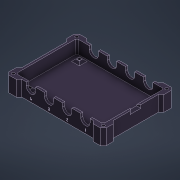
# Autodesk Inventor part: Case
Saved by Autodesk Inventor 2021.3 (Build 253353000, 353)
## iProperties
Created: 2022-02-15
Part Number: Case
Material: Generic
Document SubType Name: Modeling
Designer: Alex
Density: 1 g/cm^3
Appearance: Default
Author: Alex
Autodesk Inventor part; units mm, degrees
ref_plane "YZ Plane" through (0, 0, 0) normal (1, 0, 0) x (0, 1, 0)
ref_plane "XZ Plane" through (0, 0, 0) normal (0, 1, 0) x (-1, 0, 0)
ref_plane "XY Plane" through (0, 0, 0) normal (0, 0, 1) x (1, 0, 0)
sketch "Sketch1" plane through (0, 0, 0) normal (0, 1, 0) x (-1, 0, 0)
  line L0 (0, -45.5) -> (-50, -45.5)
  line L1 (-50, -45.5) -> (-54, -49.5)
  line L2 (-54, -49.5) -> (-64, -49.5)
  line L3 (-64, -49.5) -> (-68, -45.5)
  line L4 (-68, -45.5) -> (-68, -35.5)
  line L5 (-68, -35.5) -> (-64, -31.5)
  line L6 (-64, -31.5) -> (-64, 0)
  line L7 (0, 0) -> (0, -45.5) construction
  line L8 (0, 0) -> (-64, 0) construction
  line L9 (0, -45.5) -> (50, -45.5)
  line L10 (50, -45.5) -> (54, -49.5)
  line L11 (54, -49.5) -> (64, -49.5)
  line L12 (64, -49.5) -> (68, -45.5)
  line L13 (68, -45.5) -> (68, -35.5)
  line L14 (68, -35.5) -> (64, -31.5)
  line L15 (64, -31.5) -> (64, 0)
  line L16 (0, 0) -> (64, 0) construction
  line L17 (0, 45.5) -> (-50, 45.5)
  line L18 (-50, 45.5) -> (-54, 49.5)
  line L19 (-54, 49.5) -> (-64, 49.5)
  line L20 (-64, 49.5) -> (-68, 45.5)
  line L21 (-68, 45.5) -> (-68, 35.5)
  line L22 (-68, 35.5) -> (-64, 31.5)
  line L23 (-64, 31.5) -> (-64, 0)
  line L24 (0, 0) -> (0, 45.5) construction
  line L25 (0, 45.5) -> (50, 45.5)
  line L26 (50, 45.5) -> (54, 49.5)
  line L27 (54, 49.5) -> (64, 49.5)
  line L28 (64, 49.5) -> (68, 45.5)
  line L29 (68, 45.5) -> (68, 35.5)
  line L30 (68, 35.5) -> (64, 31.5)
  line L31 (64, 31.5) -> (64, 0)
  dimension "d6" = 100
  dimension "d7" = 10
  dimension "d10" = 135
  dimension "d11" = 4
  dimension "d22" = 91
  constraints: 64 end point, 20 symmetric about line, 3 perpendicular, 2 horizontal, 2 horizontal alignment, 2 vertical, 2 vertical alignment
  measures "d6" diameter of L0.end L7
  measures "d7" distance of L1.end L2.end
  measures "d10" angle of L0 L1
  measures "d11" distance from line of L3.end L2
  measures "d22" distance between parallel lines of L17 L0
extrude "Extrusion1" add sketch "Sketch1" along normal blind 3
sketch "Sketch2" plane through (0, 3, 0) normal (0, 1, 0) x (1, 0, 0)
  line L0 (-61, 42.5) -> (61, 42.5)
  line L1 (61, 42.5) -> (61, -42.5)
  line L2 (61, -42.5) -> (-61, -42.5)
  line L3 (-61, -42.5) -> (-61, 42.5)
  line L4 (-54, 49.5) -> (-64, 49.5) projected
  line L5 (-64, 49.5) -> (-68, 45.5) projected
  line L6 (-68, 45.5) -> (-68, 35.5) projected
  line L7 (-68, 35.5) -> (-64, 31.5) projected
  line L8 (-64, 31.5) -> (-64, -31.5) projected
  line L9 (-64, -31.5) -> (-68, -35.5) projected
  line L10 (-68, -35.5) -> (-68, -45.5) projected
  line L11 (-68, -45.5) -> (-64, -49.5) projected
  line L12 (-64, -49.5) -> (-54, -49.5) projected
  line L13 (-54, -49.5) -> (-50, -45.5) projected
  line L14 (-50, -45.5) -> (50, -45.5) projected
  line L15 (50, -45.5) -> (54, -49.5) projected
  line L16 (54, -49.5) -> (64, -49.5) projected
  line L17 (64, -49.5) -> (68, -45.5) projected
  line L18 (68, -45.5) -> (68, -35.5) projected
  line L19 (68, -35.5) -> (64, -31.5) projected
  line L20 (64, -31.5) -> (64, 31.5) projected
  line L21 (64, 31.5) -> (68, 35.5) projected
  line L22 (68, 35.5) -> (68, 45.5) projected
  line L23 (68, 45.5) -> (64, 49.5) projected
  line L24 (64, 49.5) -> (54, 49.5) projected
  line L25 (54, 49.5) -> (50, 45.5) projected
  line L26 (50, 45.5) -> (-50, 45.5) projected
  line L27 (-50, 45.5) -> (-54, 49.5) projected
  line L28 (-49.9676, 41.5746) -> (66.2374, 41.5746) construction
  line L29 (66.2374, 41.5746) -> (66.2374, -40.9754) construction
  line L30 (66.2374, -40.9754) -> (-49.9676, -40.9754) construction
  line L31 (-49.9676, -40.9754) -> (-49.9676, 41.5746) construction
  point P0 (0, 0)
  point P1 (-61, 0)
  point P2 (0, 42.5)
  dimension "d14" = 3
  dimension "d15" = 3
  dimension "d16" = 116.205
  dimension "d17" = 82.55
  constraints: 16 end point, 3 horizontal, 3 vertical, 2 midpoint, 1 horizontal alignment, 1 vertical alignment
  measures "d14" distance between parallel lines of L26 L0
  measures "d15" distance between parallel lines of L8 L3
  measures "d16" distance of L28.start L28.end
  measures "d17" distance of L30.end L28.start
extrude "Extrusion2" add sketch "Sketch2" along normal blind 18.5
sketch "Sketch4" plane through (0, 3, 0) normal (0, 1, 0) x (1, 0, 0)
  line L0 (-56.205, 41.275) -> (60, 41.275) construction
  line L1 (60, 41.275) -> (60, -41.275) construction
  line L2 (60, -41.275) -> (-56.205, -41.275) construction
  line L3 (-56.205, -41.275) -> (-56.205, 41.275) construction
  line L4 (-61, 42.5) -> (-61, -42.5) construction
  line L5 (-61, -42.5) -> (61, -42.5) construction
  line L6 (61, -42.5) -> (61, 42.5) construction
  line L7 (61, 42.5) -> (-61, 42.5) construction
  line L8 (-64, 49.5) -> (-68, 45.5) construction
  line L9 (-68, 45.5) -> (-68, 35.5) construction
  line L10 (-68, 35.5) -> (-64, 31.5) construction
  line L11 (-64, 31.5) -> (-64, -31.5) construction
  line L12 (-64, -31.5) -> (-68, -35.5) construction
  line L13 (-68, -35.5) -> (-68, -45.5) construction
  line L14 (-68, -45.5) -> (-64, -49.5) construction
  line L15 (-64, -49.5) -> (-54, -49.5) construction
  line L16 (-54, -49.5) -> (-50, -45.5) construction
  line L17 (-50, -45.5) -> (50, -45.5) construction
  line L18 (50, -45.5) -> (54, -49.5) construction
  line L19 (54, -49.5) -> (64, -49.5) construction
  line L20 (64, -49.5) -> (68, -45.5) construction
  line L21 (68, -45.5) -> (68, -35.5) construction
  line L22 (68, -35.5) -> (64, -31.5) construction
  line L23 (64, -31.5) -> (64, 31.5) construction
  line L24 (64, 31.5) -> (68, 35.5) construction
  line L25 (68, 35.5) -> (68, 45.5) construction
  line L26 (68, 45.5) -> (64, 49.5) construction
  line L27 (64, 49.5) -> (54, 49.5) construction
  line L28 (54, 49.5) -> (50, 45.5) construction
  line L29 (50, 45.5) -> (-50, 45.5) construction
  line L30 (-50, 45.5) -> (-54, 49.5) construction
  line L31 (-54, 49.5) -> (-64, 49.5) construction
  line L32 (-61, 42.5) -> (61, 42.5) construction
  line L33 (61, 42.5) -> (61, -42.5) construction
  line L34 (61, -42.5) -> (-61, -42.5) construction
  line L35 (-61, -42.5) -> (-61, 42.5) construction
  line L36 (-52.355, 37.425) -> (-47.355, 37.425)
  line L37 (-47.355, 37.425) -> (-47.355, 32.425)
  line L38 (-47.355, 32.425) -> (-52.355, 32.425)
  line L39 (-52.355, 32.425) -> (-52.355, 37.425)
  line L40 (-52.355, 37.425) -> (-47.355, 32.425) construction
  line L41 (-47.355, 37.425) -> (-52.355, 32.425) construction
  line L42 (-52.355, -32.425) -> (-52.355, -37.425)
  line L43 (-52.355, -37.425) -> (-47.355, -37.425)
  line L44 (-47.355, -37.425) -> (-47.355, -32.425)
  line L45 (-47.355, -32.425) -> (-52.355, -32.425)
  line L46 (-52.355, -32.425) -> (-47.355, -37.425) construction
  line L47 (-52.355, -37.425) -> (-47.355, -32.425) construction
  line L48 (51.15, 37.425) -> (56.15, 37.425)
  line L49 (56.15, 37.425) -> (56.15, 32.425)
  line L50 (56.15, 32.425) -> (51.15, 32.425)
  line L51 (51.15, 32.425) -> (51.15, 37.425)
  line L52 (51.15, 37.425) -> (56.15, 32.425) construction
  line L53 (56.15, 37.425) -> (51.15, 32.425) construction
  line L54 (51.15, -32.425) -> (56.15, -32.425)
  line L55 (56.15, -32.425) -> (56.15, -37.425)
  line L56 (56.15, -37.425) -> (51.15, -37.425)
  line L57 (51.15, -37.425) -> (51.15, -32.425)
  line L58 (51.15, -32.425) -> (56.15, -37.425) construction
  line L59 (56.15, -32.425) -> (51.15, -37.425) construction
  point P0 (-61, 0)
  point P1 (-56.205, 0)
  point P2 (-49.855, 34.925)
  point P3 (-49.855, -34.925)
  point P4 (53.65, 34.925)
  point P5 (53.65, -34.925)
  point P6 (-49.855, 34.925)
  point P7 (53.65, 34.925)
  point P8 (53.65, -34.925)
  point P9 (-49.855, -34.925)
  point P10 (-49.855, 34.925)
  point P11 (-49.855, -34.925)
  point P12 (53.65, -34.925)
  point P13 (53.65, 34.925)
  dimension "d20" = 116.205
  dimension "d21" = 82.55
  dimension "d23" = 6.35
  dimension "d24" = 6.35
  dimension "d25" = 6.35
  dimension "d26" = 6.35
  dimension "d27" = 5
  dimension "d28" = 1
  constraints: 56 end point, 18 midpoint, 10 horizontal, 10 vertical, 6 equal length, 3 horizontal alignment, 2 vertical alignment, 1 point on line
  measures "d20" distance of L0.start L0.end
  measures "d21" distance of L2.end L0.start
  measures "d23" distance from line of point (-49.855, 34.925) L3
  measures "d24" distance from line of point (53.65, 34.925) L1
  measures "d25" distance from line of L0 point (-49.855, 34.925)
  measures "d26" distance from line of point (-49.855, -34.925) L2
  measures "d27" distance of L36.end L37.end
  measures "d28" distance between parallel lines of L1 L6
extrude "Extrusion3" add sketch "Sketch4" along normal blind 3
chamfer "Chamfer1" distance 3 angle 45 16 edges at (-49.855, 3, -32.425) (-47.355, 3, -34.925) (-49.855, 3, -37.425) (-52.355, 3, -34.925) (53.65, 3, -32.425) (56.15, 3, -34.925) (53.65, 3, -37.425) (51.15, 3, -34.925) (53.65, 3, 32.425) (51.15, 3, 34.925) (53.65, 3, 37.425) (56.15, 3, 34.925) (-52.355, 3, 34.925) (-49.855, 3, 32.425) (-47.355, 3, 34.925) (-49.855, 3, 37.425)
sketch "Sketch5" plane through (0, 6, 0) normal (0, 1, 0) x (1, 0, 0)
  line L0 (48.15, -29.425) -> (48.15, -40.425) construction
  line L1 (59.15, -29.425) -> (48.15, -29.425) construction
  line L2 (59.15, -40.425) -> (59.15, -29.425) construction
  line L3 (48.15, -40.425) -> (59.15, -40.425) construction
  line L4 (-44.355, 29.425) -> (-44.355, 40.425) construction
  line L5 (-55.355, 29.425) -> (-44.355, 29.425) construction
  line L6 (-55.355, 40.425) -> (-55.355, 29.425) construction
  line L7 (-44.355, 40.425) -> (-55.355, 40.425) construction
  line L8 (-61, 42.5) -> (-61, -42.5) construction
  line L9 (-61, -42.5) -> (61, -42.5) construction
  line L10 (61, -42.5) -> (61, 42.5) construction
  line L11 (61, 42.5) -> (-61, 42.5) construction
  line L12 (59.15, 29.425) -> (59.15, 40.425) construction
  line L13 (48.15, 29.425) -> (59.15, 29.425) construction
  line L14 (48.15, 40.425) -> (48.15, 29.425) construction
  line L15 (59.15, 40.425) -> (48.15, 40.425) construction
  line L16 (-55.355, -29.425) -> (-55.355, -40.425) construction
  line L17 (-44.355, -29.425) -> (-55.355, -29.425) construction
  line L18 (-44.355, -40.425) -> (-44.355, -29.425) construction
  line L19 (-55.355, -40.425) -> (-44.355, -40.425) construction
  line L20 (-52.355, 32.425) -> (-47.355, 32.425) construction
  line L21 (-47.355, 32.425) -> (-47.355, 37.425) construction
  line L22 (-47.355, 37.425) -> (-52.355, 37.425) construction
  line L23 (-52.355, 37.425) -> (-52.355, 32.425) construction
  line L24 (51.15, 32.425) -> (56.15, 32.425) construction
  line L25 (56.15, 32.425) -> (56.15, 37.425) construction
  line L26 (56.15, 37.425) -> (51.15, 37.425) construction
  line L27 (51.15, 37.425) -> (51.15, 32.425) construction
  line L28 (51.15, -37.425) -> (56.15, -37.425) construction
  line L29 (56.15, -37.425) -> (56.15, -32.425) construction
  line L30 (56.15, -32.425) -> (51.15, -32.425) construction
  line L31 (51.15, -32.425) -> (51.15, -37.425) construction
  line L32 (-52.355, -37.425) -> (-47.355, -37.425) construction
  line L33 (-47.355, -37.425) -> (-47.355, -32.425) construction
  line L34 (-47.355, -32.425) -> (-52.355, -32.425) construction
  line L35 (-52.355, -32.425) -> (-52.355, -37.425) construction
  point P0 (0, 0)
  point P1 (-49.855, 34.925)
  point P2 (53.65, 34.925)
  point P3 (53.65, -34.925)
  point P4 (-49.855, -34.925)
  point P5 (-49.855, 37.425)
  point P6 (53.65, 37.425)
  point P7 (53.65, -32.425)
  point P8 (-49.855, -32.425)
  point P9 (-47.355, -34.925)
  point P10 (-47.355, 34.925)
  point P11 (56.15, 34.925)
  point P12 (56.15, -34.925)
  constraints: 8 midpoint, 4 horizontal alignment, 4 vertical alignment
hole "Hole1" at (-49.855, 6, -34.925) at (53.65, 6, -34.925) at (53.65, 6, 34.925) at (-49.855, 6, 34.925) direction (0, -1, 0) diameter 4 depth 5
sketch "Sketch6" plane through (-50, 0, 45.5) normal (0, 0, 1) x (1, 0, 0)
  line L0 (110, 3) -> (-6.205, 3) construction
  line L1 (-5.355, 3) -> (-2.355, 6) construction
  line L2 (2.645, 6) -> (5.645, 3) construction
  line L3 (-2.355, 6) -> (2.645, 6) construction
  line L4 (98.15, 3) -> (109.15, 3) construction
  line L5 (106.15, 6) -> (109.15, 3) construction
  line L6 (101.15, 6) -> (106.15, 6) construction
  line L7 (98.15, 3) -> (101.15, 6) construction
  line L8 (106.15, 6) -> (109.15, 3) construction
  line L9 (101.15, 6) -> (106.15, 6) construction
  line L10 (98.15, 3) -> (109.15, 3) construction
  line L11 (106.15, 6) -> (109.15, 3) construction
  line L12 (101.15, 6) -> (106.15, 6) construction
  line L13 (98.15, 3) -> (101.15, 6) construction
  line L14 (-1.855, 6) -> (2.145, 6) construction
  line L15 (-6.205, 7.65) -> (110, 7.65) construction
  line L16 (110, 7.65) -> (110, 6) construction
  line L17 (110, 6) -> (-6.205, 6) construction
  line L18 (-6.205, 6) -> (-6.205, 7.65) construction
  arc A0 (6.345, 16.4) -> (19.345, 16.4) centre (12.845, 16.4) ccw
  line L19 (0, 0) -> (0, 21.5) construction
  line L20 (0, 21.5) -> (100, 21.5) construction
  line L21 (100, 0) -> (100, 21.5) construction
  line L22 (0, 0) -> (100, 0) construction
  line L23 (19.345, 16.4) -> (19.345, 21.5)
  line L24 (6.345, 16.4) -> (6.345, 21.5)
  line L25 (6.345, 21.5) -> (19.345, 21.5)
  arc A1 (19.345, 16.4) -> (6.345, 16.4) centre (12.845, 16.4) ccw construction
  arc A2 (31.745, 16.4) -> (44.745, 16.4) centre (38.245, 16.4) ccw
  arc A3 (44.745, 16.4) -> (31.745, 16.4) centre (38.245, 16.4) ccw construction
  line L26 (31.745, 16.4) -> (31.745, 21.5)
  line L27 (44.745, 16.4) -> (44.745, 21.5)
  line L28 (31.745, 21.5) -> (44.745, 21.5)
  arc A4 (57.145, 16.4) -> (70.145, 16.4) centre (63.645, 16.4) ccw
  arc A5 (70.145, 16.4) -> (57.145, 16.4) centre (63.645, 16.4) ccw construction
  line L29 (57.145, 16.4) -> (57.145, 21.5)
  line L30 (70.145, 16.4) -> (70.145, 21.5)
  line L31 (57.145, 21.5) -> (70.145, 21.5)
  arc A6 (82.545, 16.4) -> (95.545, 16.4) centre (89.045, 16.4) ccw
  arc A7 (95.545, 16.4) -> (82.545, 16.4) centre (89.045, 16.4) ccw construction
  line L32 (82.545, 16.4) -> (82.545, 21.5)
  line L33 (95.545, 16.4) -> (95.545, 21.5)
  line L34 (82.545, 21.5) -> (95.545, 21.5)
  point P0 (50, 0)
  point P1 (0.145, 3)
  dimension "d41" = 1.65
  dimension "d42" = 116.205
  dimension "d43" = 6.35
  dimension "d44" = 13
  dimension "d46" = 12.7
  dimension "d49" = 25.4
  dimension "d71" = 10.4
  constraints: 32 end point, 16 point on circle, 8 centre point, 4 horizontal, 4 vertical, 2 collinear, 2 tangent, 30 other
  measures "d41" distance of L15.end L16.end
  measures "d42" distance of L16.end L17.end
  measures "d43" distance from line of point (0.145, 3) L18
  measures "d44" diameter of A0
  measures "d46" horizontal distance of A0.centre point (0.145, 3)
  measures "d49" distance of L24.start L26.start
  measures "d71" distance from line of L17 A0.centre
extrude "Extrusion4" cut sketch "Sketch6" against normal through all
chamfer "Chamfer2" distance 2 angle 45 4 edges at (-61, 12.25, -42.5) (-61, 12.25, 42.5) (61, 12.25, 42.5) (61, 12.25, -42.5)
sketch "Sketch7" plane through (0, 21.5, 0) normal (0, 1, 0) x (1, 0, 0)
  line L0 (-43.655, -45.5) -> (-43.655, -42.5) construction
  line L1 (-43.655, -42.5) -> (-59, -42.5) construction
  line L2 (-61, -40.5) -> (-59, -42.5) construction
  line L3 (-61, -40.5) -> (-61, 40.5) construction
  line L4 (-59, 42.5) -> (-61, 40.5) construction
  line L5 (-59, 42.5) -> (-43.655, 42.5) construction
  line L6 (-43.655, 42.5) -> (-43.655, 45.5) construction
  line L7 (-43.655, 45.5) -> (-50, 45.5) construction
  line L8 (-50, 45.5) -> (-54, 49.5) construction
  line L9 (-54, 49.5) -> (-64, 49.5) construction
  line L10 (-64, 49.5) -> (-68, 45.5) construction
  line L11 (-68, 45.5) -> (-68, 35.5) construction
  line L12 (-68, 35.5) -> (-64, 31.5) construction
  line L13 (-64, 31.5) -> (-64, -31.5) construction
  line L14 (-64, -31.5) -> (-68, -35.5) construction
  line L15 (-68, -35.5) -> (-68, -45.5) construction
  line L16 (-68, -45.5) -> (-64, -49.5) construction
  line L17 (-64, -49.5) -> (-54, -49.5) construction
  line L18 (-54, -49.5) -> (-50, -45.5) construction
  line L19 (-50, -45.5) -> (-43.655, -45.5) construction
  line L20 (45.545, -42.5) -> (45.545, -45.5) construction
  line L21 (45.545, -45.5) -> (50, -45.5) construction
  line L22 (50, -45.5) -> (54, -49.5) construction
  line L23 (54, -49.5) -> (64, -49.5) construction
  line L24 (64, -49.5) -> (68, -45.5) construction
  line L25 (68, -45.5) -> (68, -35.5) construction
  line L26 (68, -35.5) -> (64, -31.5) construction
  line L27 (64, -31.5) -> (64, 31.5) construction
  line L28 (64, 31.5) -> (68, 35.5) construction
  line L29 (68, 35.5) -> (68, 45.5) construction
  line L30 (68, 45.5) -> (64, 49.5) construction
  line L31 (64, 49.5) -> (54, 49.5) construction
  line L32 (54, 49.5) -> (50, 45.5) construction
  line L33 (50, 45.5) -> (45.545, 45.5) construction
  line L34 (45.545, 45.5) -> (45.545, 42.5) construction
  line L35 (45.545, 42.5) -> (59, 42.5) construction
  line L36 (61, 40.5) -> (59, 42.5) construction
  line L37 (61, 40.5) -> (61, -40.5) construction
  line L38 (59, -42.5) -> (61, -40.5) construction
  line L39 (59, -42.5) -> (45.545, -42.5) construction
  point P0 (0, 0)
  point P1 (-63, 44.5)
  point P2 (-63, -44.5)
  point P3 (63, -44.5)
  point P4 (63, 44.5)
  dimension "d59" = 5
  dimension "d60" = 5
  dimension "d61" = 5
  dimension "d62" = 5
  constraints: 2 horizontal alignment, 2 vertical alignment
  measures "d59" distance from line of L11 point (-63, 44.5)
  measures "d60" distance from line of point (-63, 44.5) L9
  measures "d61" distance from line of point (-63, -44.5) L17
  measures "d62" distance from line of L29 point (63, 44.5)
hole "Hole2" at (-63, 21.5, -44.5) at (-63, 21.5, 44.5) at (63, 21.5, 44.5) at (63, 21.5, -44.5) direction (0, -1, 0) diameter 4 depth 5
sketch "Sketch8" plane through (-50, 0, 45.5) normal (0, 0, 1) x (1, 0, 0)
  line L0 (10.345, 6.9) -> (15.345, 6.9) construction
  line L1 (15.345, 6.9) -> (15.345, 1.9) construction
  line L2 (15.345, 1.9) -> (10.345, 1.9) construction
  line L3 (10.345, 1.9) -> (10.345, 6.9) construction
  line L4 (35.745, 6.9) -> (40.745, 6.9) construction
  line L5 (40.745, 6.9) -> (40.745, 1.9) construction
  line L6 (40.745, 1.9) -> (35.745, 1.9) construction
  line L7 (35.745, 1.9) -> (35.745, 6.9) construction
  line L8 (61.145, 6.9) -> (66.145, 6.9) construction
  line L9 (66.145, 6.9) -> (66.145, 1.9) construction
  line L10 (66.145, 1.9) -> (61.145, 1.9) construction
  line L11 (61.145, 1.9) -> (61.145, 6.9) construction
  line L12 (86.545, 6.9) -> (91.545, 6.9) construction
  line L13 (91.545, 6.9) -> (91.545, 1.9) construction
  line L14 (91.545, 1.9) -> (86.545, 1.9) construction
  line L15 (86.545, 1.9) -> (86.545, 6.9) construction
  line L16 (57.145, 16.4) -> (57.145, 21.5) construction
  line L17 (44.745, 21.5) -> (57.145, 21.5) construction
  line L18 (44.745, 21.5) -> (44.745, 16.4) construction
  arc A0 (31.745, 16.4) -> (44.745, 16.4) centre (38.245, 16.4) ccw construction
  line L19 (31.745, 16.4) -> (31.745, 21.5) construction
  line L20 (19.345, 21.5) -> (31.745, 21.5) construction
  line L21 (19.345, 21.5) -> (19.345, 16.4) construction
  arc A1 (6.345, 16.4) -> (19.345, 16.4) centre (12.845, 16.4) ccw construction
  line L22 (6.345, 16.4) -> (6.345, 21.5) construction
  line L23 (0, 21.5) -> (6.345, 21.5) construction
  line L24 (0, 0) -> (0, 21.5) construction
  line L25 (0, 0) -> (100, 0) construction
  line L26 (100, 0) -> (100, 21.5) construction
  line L27 (95.545, 21.5) -> (100, 21.5) construction
  line L28 (95.545, 21.5) -> (95.545, 16.4) construction
  arc A2 (82.545, 16.4) -> (95.545, 16.4) centre (89.045, 16.4) ccw construction
  line L29 (82.545, 16.4) -> (82.545, 21.5) construction
  line L30 (70.145, 21.5) -> (82.545, 21.5) construction
  line L31 (70.145, 21.5) -> (70.145, 16.4) construction
  arc A3 (57.145, 16.4) -> (70.145, 16.4) centre (63.645, 16.4) ccw construction
  line L32 (13.8281, 3.2125) -> (13.4779, 3.2125)
  line L33 (13.4779, 3.2125) -> (13.4779, 2.8119)
  spline S0 degree 2 poles (13.4779, 2.8119) (13.4779, 2.65) (13.3213, 2.65) knots 0 0 0 1 1 1
  spline S1 degree 2 poles (13.3213, 2.65) (13.1621, 2.65) (13.1621, 2.8119) knots 0 0 0 1 1 1
  line L34 (13.1621, 2.8119) -> (13.1621, 3.2125)
  line L35 (13.1621, 3.2125) -> (11.5726, 3.2125)
  spline S2 degree 2 poles (11.5726, 3.2125) (11.4771, 3.2125) (11.4771, 3.3505) knots 0 0 0 1 1 1
  spline S3 degree 2 poles (11.4771, 3.3505) (11.4771, 3.4461) (11.5169, 3.5575) knots 0 0 0 1 1 1
  line L36 (11.5169, 3.5575) -> (12.3873, 6.0412)
  spline S4 degree 2 poles (12.3873, 6.0412) (12.4218, 6.15) (12.5279, 6.15) knots 0 0 0 1 1 1
  spline S5 degree 2 poles (12.5279, 6.15) (12.5942, 6.15) (12.6951, 6.0571) (12.6951, 5.9908) knots 0 0 0 1 2 2 2
  spline S6 degree 2 poles (12.6951, 5.9908) (12.6951, 5.9669) (12.6871, 5.9351) knots 0 0 0 1 1 1
  line L37 (12.6871, 5.9351) -> (11.8513, 3.5336)
  line L38 (11.8513, 3.5336) -> (13.1621, 3.5336)
  line L39 (13.1621, 3.5336) -> (13.1621, 4.205)
  spline S7 degree 2 poles (13.1621, 4.205) (13.1621, 4.3668) (13.3213, 4.3668) knots 0 0 0 1 1 1
  spline S8 degree 2 poles (13.3213, 4.3668) (13.4779, 4.3668) (13.4779, 4.205) knots 0 0 0 1 1 1
  line L40 (13.4779, 4.205) -> (13.4779, 3.5336)
  line L41 (13.4779, 3.5336) -> (13.8308, 3.5336)
  spline S9 degree 2 poles (13.8308, 3.5336) (13.99, 3.5336) (13.99, 3.3744) knots 0 0 0 1 1 1
  spline S10 degree 2 poles (13.99, 3.3744) (13.99, 3.2125) (13.8281, 3.2125) knots 0 0 0 1 1 1
  spline S11 degree 2 poles (39.2149, 3.9502) (39.2149, 3.263) (38.7425, 2.918) knots 0 0 0 1 1 1
  spline S12 degree 2 poles (38.7425, 2.918) (38.2994, 2.5996) (37.782, 2.7561) knots 0 0 0 1 1 1
  spline S13 degree 2 poles (37.782, 2.7561) (37.2353, 2.9233) (37.0416, 3.523) knots 0 0 0 1 1 1
  spline S14 degree 2 poles (37.0416, 3.523) (37.031, 3.5549) (37.031, 3.5787) knots 0 0 0 1 1 1
  spline S15 degree 2 poles (37.031, 3.5787) (37.031, 3.7273) (37.1876, 3.7273) knots 0 0 0 1 1 1
  spline S16 degree 2 poles (37.1876, 3.7273) (37.2964, 3.7273) (37.3309, 3.6185) knots 0 0 0 1 1 1
  spline S17 degree 2 poles (37.3309, 3.6185) (37.4211, 3.3346) (37.6413, 3.1834) knots 0 0 0 1 1 1
  spline S18 degree 2 poles (37.6413, 3.1834) (37.8377, 3.0401) (38.0871, 3.0401) knots 0 0 0 1 1 1
  spline S19 degree 2 poles (38.0871, 3.0401) (38.4162, 3.0401) (38.6497, 3.2736) knots 0 0 0 1 1 1
  spline S20 degree 2 poles (38.6497, 3.2736) (38.9097, 3.5283) (38.9097, 3.9502) knots 0 0 0 1 1 1
  spline S21 degree 2 poles (38.9097, 3.9502) (38.9097, 4.3907) (38.647, 4.6189) knots 0 0 0 1 1 1
  spline S22 degree 2 poles (38.647, 4.6189) (38.4533, 4.7887) (38.1269, 4.8392) knots 0 0 0 1 1 1
  spline S23 degree 2 poles (38.1269, 4.8392) (37.9544, 4.8498) (37.6201, 4.8843) (37.6201, 4.9745) knots 0 0 0 1 2 2 2
  spline S24 degree 2 poles (37.6201, 4.9745) (37.6201, 5.0567) (37.697, 5.1337) knots 0 0 0 1 1 1
  line L42 (37.697, 5.1337) -> (38.4321, 5.8793)
  line L43 (38.4321, 5.8793) -> (37.3468, 5.8793)
  spline S25 degree 2 poles (37.3468, 5.8793) (37.1876, 5.8793) (37.1876, 6.0386) knots 0 0 0 1 1 1
  spline S26 degree 2 poles (37.1876, 6.0386) (37.1876, 6.1951) (37.3468, 6.1951) knots 0 0 0 1 1 1
  line L44 (37.3468, 6.1951) -> (38.9044, 6.2004)
  spline S27 degree 2 poles (38.9044, 6.2004) (39.0265, 6.2004) (39.0265, 6.1208) knots 0 0 0 1 1 1
  spline S28 degree 2 poles (39.0265, 6.1208) (39.0265, 6.0545) (38.8779, 5.9032) knots 0 0 0 1 1 1
  line L45 (38.8779, 5.9032) -> (38.1641, 5.1629)
  spline S29 degree 2 poles (38.1641, 5.1629) (39.2149, 5.0223) (39.2149, 3.9502) knots 0 0 0 1 1 1
  line L46 (64.4238, 2.6659) -> (62.4894, 2.6659)
  spline S30 degree 2 poles (62.4894, 2.6659) (62.577, 2.987) (62.6619, 3.3001) knots 0 0 0 1 1 1
  spline S31 degree 2 poles (62.6619, 3.3001) (62.7999, 3.7273) (63.044, 4.0404) knots 0 0 0 1 1 1
  spline S32 degree 2 poles (63.044, 4.0404) (63.3677, 4.4571) (63.9382, 4.7781) knots 0 0 0 1 1 1
  spline S33 degree 2 poles (63.9382, 4.7781) (64.2832, 4.9692) (64.2832, 5.3062) knots 0 0 0 1 1 1
  spline S34 degree 2 poles (64.2832, 5.3062) (64.2832, 5.5132) (64.1346, 5.6618) knots 0 0 0 1 1 1
  spline S35 degree 2 poles (64.1346, 5.6618) (63.9727, 5.813) (63.71, 5.813) knots 0 0 0 1 1 1
  spline S36 degree 2 poles (63.71, 5.813) (63.4181, 5.813) (63.2563, 5.7281) knots 0 0 0 1 1 1
  spline S37 degree 2 poles (63.2563, 5.7281) (63.0679, 5.6193) (62.9564, 5.346) knots 0 0 0 1 1 1
  spline S38 degree 2 poles (62.9564, 5.346) (62.9166, 5.2505) (62.8237, 5.2505) knots 0 0 0 1 1 1
  spline S39 degree 2 poles (62.8237, 5.2505) (62.6672, 5.2505) (62.6672, 5.4044) knots 0 0 0 1 1 1
  spline S40 degree 2 poles (62.6672, 5.4044) (62.6672, 5.4335) (62.6831, 5.468) knots 0 0 0 1 1 1
  spline S41 degree 2 poles (62.6831, 5.468) (62.9564, 6.1341) (63.6888, 6.1341) knots 0 0 0 1 1 1
  spline S42 degree 2 poles (63.6888, 6.1341) (64.1187, 6.1341) (64.3787, 5.89) knots 0 0 0 1 1 1
  spline S43 degree 2 poles (64.3787, 5.89) (64.6175, 5.6671) (64.6175, 5.3327) knots 0 0 0 1 1 1
  spline S44 degree 2 poles (64.6175, 5.3327) (64.6175, 4.81) (64.0842, 4.5048) knots 0 0 0 1 1 1
  spline S45 degree 2 poles (64.0842, 4.5048) (63.4606, 4.1492) (63.1793, 3.6928) knots 0 0 0 1 1 1
  spline S46 degree 2 poles (63.1793, 3.6928) (63.044, 3.4646) (62.9113, 2.9817) knots 0 0 0 1 1 1
  line L47 (62.9113, 2.9817) -> (64.4238, 2.9817)
  spline S47 degree 2 poles (64.4238, 2.9817) (64.583, 2.9817) (64.583, 2.8251) knots 0 0 0 1 1 1
  spline S48 degree 2 poles (64.583, 2.8251) (64.583, 2.6659) (64.4238, 2.6659) knots 0 0 0 1 1 1
  spline S49 degree 2 poles (89.1538, 2.8145) (89.1538, 2.658) (88.9999, 2.658) knots 0 0 0 1 1 1
  spline S50 degree 2 poles (88.9999, 2.658) (88.8433, 2.658) (88.8433, 2.8145) knots 0 0 0 1 1 1
  line L48 (88.8433, 2.8145) -> (88.8433, 5.9855)
  spline S51 degree 2 poles (88.8433, 5.9855) (88.8433, 6.142) (88.9999, 6.142) knots 0 0 0 1 1 1
  spline S52 degree 2 poles (88.9999, 6.142) (89.1538, 6.142) (89.1538, 5.9855) knots 0 0 0 1 1 1
  line L49 (89.1538, 5.9855) -> (89.1538, 2.8145)
  point P0 (50, 0)
  point P1 (38.245, 9.9)
  point P2 (38.245, 6.9)
  point P3 (63.645, 6.9)
  point P4 (63.645, 9.9)
  point P5 (89.045, 6.9)
  point P6 (89.045, 9.9)
  point P7 (12.845, 9.9)
  point P8 (12.845, 6.9)
  point P9 (15.345, 4.4)
  dimension "d72" = 5
  dimension "d74" = 3
  constraints: 6 collinear, 5 midpoint, 5 vertical alignment, 4 equal length, 4 point on circle, 1 horizontal, 8 other
  measures "d72" distance of L1.end L2.end
  measures "d74" distance of point (12.845, 6.9) point (12.845, 9.9)
emboss "Emboss1" sketch "Sketch8" operation cut depth 1 direction (0, 0, -1)
sketch "Sketch9" plane through (50, 0, -45.5) normal (0, 0, -1) x (-1, 0, 0)
  line L0 (42.855, 21.5) -> (42.855, 16.4) construction
  arc A0 (29.855, 16.4) -> (42.855, 16.4) centre (36.355, 16.4) ccw construction
  line L1 (29.855, 16.4) -> (29.855, 21.5) construction
  line L2 (17.455, 21.5) -> (29.855, 21.5) construction
  line L3 (17.455, 21.5) -> (17.455, 16.4) construction
  arc A1 (4.455, 16.4) -> (17.455, 16.4) centre (10.955, 16.4) ccw construction
  line L4 (4.455, 16.4) -> (4.455, 21.5) construction
  line L5 (0, 21.5) -> (4.455, 21.5) construction
  line L6 (0, 0) -> (0, 21.5) construction
  line L7 (0, 0) -> (100, 0) construction
  line L8 (100, 0) -> (100, 21.5) construction
  line L9 (93.655, 21.5) -> (100, 21.5) construction
  line L10 (93.655, 21.5) -> (93.655, 16.4) construction
  arc A2 (80.655, 16.4) -> (93.655, 16.4) centre (87.155, 16.4) ccw construction
  line L11 (80.655, 16.4) -> (80.655, 21.5) construction
  line L12 (68.255, 21.5) -> (80.655, 21.5) construction
  line L13 (68.255, 21.5) -> (68.255, 16.4) construction
  arc A3 (55.255, 16.4) -> (68.255, 16.4) centre (61.755, 16.4) ccw construction
  line L14 (55.255, 16.4) -> (55.255, 21.5) construction
  line L15 (42.855, 21.5) -> (55.255, 21.5) construction
  line L16 (8.455, 6.9) -> (13.455, 6.9) construction
  line L17 (13.455, 6.9) -> (13.455, 1.9) construction
  line L18 (13.455, 1.9) -> (8.455, 1.9) construction
  line L19 (8.455, 1.9) -> (8.455, 6.9) construction
  line L20 (33.855, 6.9) -> (38.855, 6.9) construction
  line L21 (38.855, 6.9) -> (38.855, 1.9) construction
  line L22 (38.855, 1.9) -> (33.855, 1.9) construction
  line L23 (33.855, 1.9) -> (33.855, 6.9) construction
  line L24 (59.255, 6.9) -> (64.255, 6.9) construction
  line L25 (64.255, 6.9) -> (64.255, 1.9) construction
  line L26 (64.255, 1.9) -> (59.255, 1.9) construction
  line L27 (59.255, 1.9) -> (59.255, 6.9) construction
  line L28 (84.655, 6.9) -> (89.655, 6.9) construction
  line L29 (89.655, 6.9) -> (89.655, 1.9) construction
  line L30 (89.655, 1.9) -> (84.655, 1.9) construction
  line L31 (84.655, 1.9) -> (84.655, 6.9) construction
  spline S0 degree 2 poles (11.0638, 2.8145) (11.0638, 2.658) (10.9099, 2.658) knots 0 0 0 1 1 1
  spline S1 degree 2 poles (10.9099, 2.658) (10.7533, 2.658) (10.7533, 2.8145) knots 0 0 0 1 1 1
  line L32 (10.7533, 2.8145) -> (10.7533, 5.9855)
  spline S2 degree 2 poles (10.7533, 5.9855) (10.7533, 6.142) (10.9099, 6.142) knots 0 0 0 1 1 1
  spline S3 degree 2 poles (10.9099, 6.142) (11.0638, 6.142) (11.0638, 5.9855) knots 0 0 0 1 1 1
  line L33 (11.0638, 5.9855) -> (11.0638, 2.8145)
  line L34 (37.1338, 2.6659) -> (35.1994, 2.6659)
  spline S4 degree 2 poles (35.1994, 2.6659) (35.287, 2.987) (35.3719, 3.3001) knots 0 0 0 1 1 1
  spline S5 degree 2 poles (35.3719, 3.3001) (35.5099, 3.7273) (35.754, 4.0404) knots 0 0 0 1 1 1
  spline S6 degree 2 poles (35.754, 4.0404) (36.0777, 4.4571) (36.6482, 4.7781) knots 0 0 0 1 1 1
  spline S7 degree 2 poles (36.6482, 4.7781) (36.9932, 4.9692) (36.9932, 5.3062) knots 0 0 0 1 1 1
  spline S8 degree 2 poles (36.9932, 5.3062) (36.9932, 5.5132) (36.8446, 5.6618) knots 0 0 0 1 1 1
  spline S9 degree 2 poles (36.8446, 5.6618) (36.6827, 5.813) (36.42, 5.813) knots 0 0 0 1 1 1
  spline S10 degree 2 poles (36.42, 5.813) (36.1281, 5.813) (35.9663, 5.7281) knots 0 0 0 1 1 1
  spline S11 degree 2 poles (35.9663, 5.7281) (35.7779, 5.6193) (35.6664, 5.346) knots 0 0 0 1 1 1
  spline S12 degree 2 poles (35.6664, 5.346) (35.6266, 5.2505) (35.5337, 5.2505) knots 0 0 0 1 1 1
  spline S13 degree 2 poles (35.5337, 5.2505) (35.3772, 5.2505) (35.3772, 5.4044) knots 0 0 0 1 1 1
  spline S14 degree 2 poles (35.3772, 5.4044) (35.3772, 5.4335) (35.3931, 5.468) knots 0 0 0 1 1 1
  spline S15 degree 2 poles (35.3931, 5.468) (35.6664, 6.1341) (36.3988, 6.1341) knots 0 0 0 1 1 1
  spline S16 degree 2 poles (36.3988, 6.1341) (36.8287, 6.1341) (37.0887, 5.89) knots 0 0 0 1 1 1
  spline S17 degree 2 poles (37.0887, 5.89) (37.3275, 5.6671) (37.3275, 5.3327) knots 0 0 0 1 1 1
  spline S18 degree 2 poles (37.3275, 5.3327) (37.3275, 4.81) (36.7942, 4.5048) knots 0 0 0 1 1 1
  spline S19 degree 2 poles (36.7942, 4.5048) (36.1706, 4.1492) (35.8893, 3.6928) knots 0 0 0 1 1 1
  spline S20 degree 2 poles (35.8893, 3.6928) (35.754, 3.4646) (35.6213, 2.9817) knots 0 0 0 1 1 1
  line L35 (35.6213, 2.9817) -> (37.1338, 2.9817)
  spline S21 degree 2 poles (37.1338, 2.9817) (37.293, 2.9817) (37.293, 2.8251) knots 0 0 0 1 1 1
  spline S22 degree 2 poles (37.293, 2.8251) (37.293, 2.6659) (37.1338, 2.6659) knots 0 0 0 1 1 1
  spline S23 degree 2 poles (62.7249, 3.9502) (62.7249, 3.263) (62.2525, 2.918) knots 0 0 0 1 1 1
  spline S24 degree 2 poles (62.2525, 2.918) (61.8094, 2.5996) (61.292, 2.7561) knots 0 0 0 1 1 1
  spline S25 degree 2 poles (61.292, 2.7561) (60.7453, 2.9233) (60.5516, 3.523) knots 0 0 0 1 1 1
  spline S26 degree 2 poles (60.5516, 3.523) (60.541, 3.5549) (60.541, 3.5787) knots 0 0 0 1 1 1
  spline S27 degree 2 poles (60.541, 3.5787) (60.541, 3.7273) (60.6976, 3.7273) knots 0 0 0 1 1 1
  spline S28 degree 2 poles (60.6976, 3.7273) (60.8064, 3.7273) (60.8409, 3.6185) knots 0 0 0 1 1 1
  spline S29 degree 2 poles (60.8409, 3.6185) (60.9311, 3.3346) (61.1513, 3.1834) knots 0 0 0 1 1 1
  spline S30 degree 2 poles (61.1513, 3.1834) (61.3477, 3.0401) (61.5971, 3.0401) knots 0 0 0 1 1 1
  spline S31 degree 2 poles (61.5971, 3.0401) (61.9262, 3.0401) (62.1597, 3.2736) knots 0 0 0 1 1 1
  spline S32 degree 2 poles (62.1597, 3.2736) (62.4197, 3.5283) (62.4197, 3.9502) knots 0 0 0 1 1 1
  spline S33 degree 2 poles (62.4197, 3.9502) (62.4197, 4.3907) (62.157, 4.6189) knots 0 0 0 1 1 1
  spline S34 degree 2 poles (62.157, 4.6189) (61.9633, 4.7887) (61.6369, 4.8392) knots 0 0 0 1 1 1
  spline S35 degree 2 poles (61.6369, 4.8392) (61.4644, 4.8498) (61.1301, 4.8843) (61.1301, 4.9745) knots 0 0 0 1 2 2 2
  spline S36 degree 2 poles (61.1301, 4.9745) (61.1301, 5.0567) (61.207, 5.1337) knots 0 0 0 1 1 1
  line L36 (61.207, 5.1337) -> (61.9421, 5.8793)
  line L37 (61.9421, 5.8793) -> (60.8568, 5.8793)
  spline S37 degree 2 poles (60.8568, 5.8793) (60.6976, 5.8793) (60.6976, 6.0386) knots 0 0 0 1 1 1
  spline S38 degree 2 poles (60.6976, 6.0386) (60.6976, 6.1951) (60.8568, 6.1951) knots 0 0 0 1 1 1
  line L38 (60.8568, 6.1951) -> (62.4144, 6.2004)
  spline S39 degree 2 poles (62.4144, 6.2004) (62.5365, 6.2004) (62.5365, 6.1208) knots 0 0 0 1 1 1
  spline S40 degree 2 poles (62.5365, 6.1208) (62.5365, 6.0545) (62.3879, 5.9032) knots 0 0 0 1 1 1
  line L39 (62.3879, 5.9032) -> (61.6741, 5.1629)
  spline S41 degree 2 poles (61.6741, 5.1629) (62.7249, 5.0223) (62.7249, 3.9502) knots 0 0 0 1 1 1
  line L40 (88.1381, 3.2125) -> (87.7879, 3.2125)
  line L41 (87.7879, 3.2125) -> (87.7879, 2.8119)
  spline S42 degree 2 poles (87.7879, 2.8119) (87.7879, 2.65) (87.6313, 2.65) knots 0 0 0 1 1 1
  spline S43 degree 2 poles (87.6313, 2.65) (87.4721, 2.65) (87.4721, 2.8119) knots 0 0 0 1 1 1
  line L42 (87.4721, 2.8119) -> (87.4721, 3.2125)
  line L43 (87.4721, 3.2125) -> (85.8826, 3.2125)
  spline S44 degree 2 poles (85.8826, 3.2125) (85.7871, 3.2125) (85.7871, 3.3505) knots 0 0 0 1 1 1
  spline S45 degree 2 poles (85.7871, 3.3505) (85.7871, 3.4461) (85.8269, 3.5575) knots 0 0 0 1 1 1
  line L44 (85.8269, 3.5575) -> (86.6973, 6.0412)
  spline S46 degree 2 poles (86.6973, 6.0412) (86.7318, 6.15) (86.8379, 6.15) knots 0 0 0 1 1 1
  spline S47 degree 2 poles (86.8379, 6.15) (86.9042, 6.15) (87.0051, 6.0571) (87.0051, 5.9908) knots 0 0 0 1 2 2 2
  spline S48 degree 2 poles (87.0051, 5.9908) (87.0051, 5.9669) (86.9971, 5.9351) knots 0 0 0 1 1 1
  line L45 (86.9971, 5.9351) -> (86.1613, 3.5336)
  line L46 (86.1613, 3.5336) -> (87.4721, 3.5336)
  line L47 (87.4721, 3.5336) -> (87.4721, 4.205)
  spline S49 degree 2 poles (87.4721, 4.205) (87.4721, 4.3668) (87.6313, 4.3668) knots 0 0 0 1 1 1
  spline S50 degree 2 poles (87.6313, 4.3668) (87.7879, 4.3668) (87.7879, 4.205) knots 0 0 0 1 1 1
  line L48 (87.7879, 4.205) -> (87.7879, 3.5336)
  line L49 (87.7879, 3.5336) -> (88.1408, 3.5336)
  spline S51 degree 2 poles (88.1408, 3.5336) (88.3, 3.5336) (88.3, 3.3744) knots 0 0 0 1 1 1
  spline S52 degree 2 poles (88.3, 3.3744) (88.3, 3.2125) (88.1381, 3.2125) knots 0 0 0 1 1 1
  point P0 (50, 0)
  point P1 (10.955, 6.9)
  point P2 (10.955, 9.9)
  point P3 (36.355, 6.9)
  point P4 (36.355, 9.9)
  point P5 (61.755, 6.9)
  point P6 (61.755, 9.9)
  point P7 (87.155, 6.9)
  point P8 (87.155, 9.9)
  dimension "d77" = 5
  dimension "d79" = 3
  constraints: 7 equal length, 6 collinear, 4 midpoint, 4 point on circle, 4 vertical alignment, 1 horizontal, 8 other
  measures "d77" distance of L18.end L16.start
  measures "d79" distance from line of L16 point (10.955, 9.9)
emboss "Emboss2" sketch "Sketch9" operation cut depth 1 direction (0, 0, 1)
sketch "Sketch10" plane through (64, 0, 31.5) normal (1, 0, 0) x (0, 0, -1)
  line L0 (0, 0) -> (63, 0) construction
  line L1 (63, 0) -> (63, 21.5) construction
  line L2 (0, 21.5) -> (63, 21.5) construction
  line L3 (0, 0) -> (0, 21.5) construction
  line L4 (72, 3) -> (72, 21.5) construction
  line L5 (-9, 3) -> (72, 3) construction
  line L6 (-9, 21.5) -> (-9, 3) construction
  line L7 (72, 21.5) -> (-9, 21.5) construction
  line L8 (-8.925, 3) -> (2.075, 3) construction
  line L9 (-0.925, 6) -> (2.075, 3) construction
  line L10 (-5.925, 6) -> (-0.925, 6) construction
  line L11 (-5.925, 6) -> (-8.925, 3) construction
  line L12 (63.925, 6) -> (68.925, 6) construction
  line L13 (63.925, 6) -> (60.925, 3) construction
  line L14 (60.925, 3) -> (71.925, 3) construction
  line L15 (68.925, 6) -> (71.925, 3) construction
  line L16 (26.725, 25) -> (35.725, 25)
  line L17 (35.725, 25) -> (35.725, 20)
  line L18 (35.725, 20) -> (26.725, 20)
  line L19 (26.725, 20) -> (26.725, 25)
  point P0 (31.5, 0)
  point P1 (-9.775, 3)
  point P2 (-9.775, 3)
  point P3 (-9.775, 3)
  dimension "d83" = 5
  dimension "d84" = 14
  dimension "d85" = 9
  dimension "d86" = 36.5
  constraints: 8 end point, 2 vertical, 1 horizontal
  measures "d83" distance of L16.end L17.end
  measures "d84" distance between parallel lines of L18 L10
  measures "d85" distance of L16.start L16.end
  measures "d86" distance from line of L19 point (-9.775, 3)
extrude "Extrusion5" cut sketch "Sketch10" against normal blind 10
chamfer "Chamfer3" distance 3 angle 45 3 edges at (64, 20, 0.275) (64, 20.75, 4.775) (64, 20.75, -4.225)
equation "\"d15\" = d14"
equation "\"d24\" = d23"
equation "\"d25\" = d23"
equation "\"d26\" = d23"
body "Solid1"
